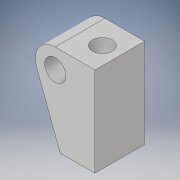
# Autodesk Inventor part: Federgelenkblock
Saved by Autodesk Inventor 2019 (Build 230136000, 136)
## iProperties
Created: 2022-03-15
Part Number: Federgelenkblock
Material: Generic
Document SubType Name: Modeling
Designer: Lukas
Density: 1 g/cm^3
Appearance: Default
Author: Lukas
Autodesk Inventor part; units mm, degrees
ref_plane "YZ Plane" through (0, 0, 0) normal (1, 0, 0) x (0, 1, 0)
ref_plane "XZ Plane" through (0, 0, 0) normal (0, 1, 0) x (-1, 0, 0)
ref_plane "XY Plane" through (0, 0, 0) normal (0, 0, 1) x (1, 0, 0)
sketch "Sketch1" plane through (0, 0, 0) normal (0, 0, 1) x (1, 0, 0)
  arc A0 (0, 4) -> (-3.7432, -1.4102) centre (0, 0) ccw
  line L0 (0, 4) -> (8, 4)
  line L1 (8, 4) -> (8, -14)
  line L2 (8, -14) -> (1, -14)
  line L3 (1, -14) -> (-3.7432, -1.4102)
  circle A1 centre (0, 0) radius 2.15
  dimension "d0" = 4
  dimension "d1" = 4.3
  dimension "d2" = 8
  dimension "d3" = 18
  dimension "d4" = 7
  constraints: 8 end point, 2 centre point, 2 coincident, 2 horizontal, 2 point on circle, 2 tangent, 1 vertical
  measures "d0" radius of A0
  measures "d1" diameter of A1
  measures "d2" distance from line of L1 point (0, 0)
  measures "d3" distance of L0.end L1.end
  measures "d4" distance of L1.end L2.end
extrude "Extrusion1" add sketch "Sketch1" along normal blind 10
sketch "Sketch2" plane through (0, 4, 0) normal (0, 1, 0) x (1, 0, 0)
  circle A0 centre (4.5, -5) radius 2
  line L0 (2.15, -10) -> (-2.15, -10) projected
  line L1 (-2.15, 0) -> (2.15, 0) projected
  line L2 (2.15, 0) -> (2.15, -10) projected
  line L3 (-2.15, 0) -> (-2.15, -10) projected
  line L4 (8, 0) -> (8, -10) projected
  line L5 (8, 0) -> (8, -10) projected
  point P0 (0, 0)
  point P1 (8, -5)
  dimension "d7" = 3.5
  dimension "d8" = 4
  constraints: 1 centre point, 1 horizontal alignment, 1 midpoint
  measures "d7" distance from line of L4 A0.centre
  measures "d8" diameter of A0
extrude "Extrusion2" cut sketch "Sketch2" against normal through all contours A0
body "Solid1"
